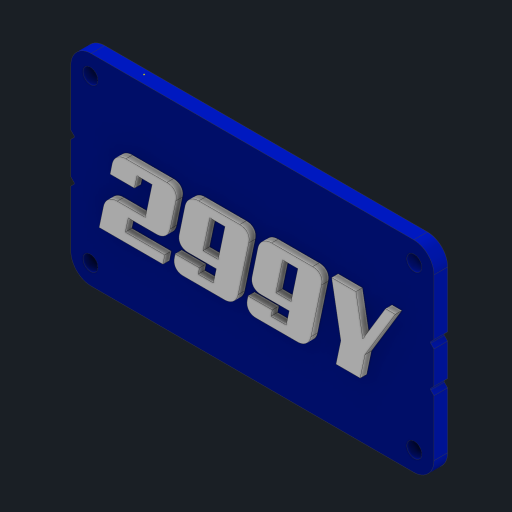
# Autodesk Inventor part: 299Y
Saved by Autodesk Inventor 2023 (Build 270158000, 158)
## iProperties
Created: 2023-05-30
Part Number: 299Y
Material: Generic
Document SubType Name: Modeling
Designer: reima
Density: 1 g/cm^3
Appearance: Default
Author: reima
Autodesk Inventor part; units mm, degrees
ref_plane "YZ Plane" through (0, 0, 0) normal (1, 0, 0) x (0, 1, 0)
ref_plane "XZ Plane" through (0, 0, 0) normal (0, 1, 0) x (-1, 0, 0)
ref_plane "XY Plane" through (0, 0, 0) normal (0, 0, 1) x (1, 0, 0)
sketch "Sketch1" plane through (0, 0, 0) normal (0, 0, 1) x (1, 0, 0)
  circle A0 centre (-16.8236, -8.8233) radius 2.1 projected
  circle A1 centre (84.7764, -8.8233) radius 2.1 projected
  circle A2 centre (84.7764, -59.6233) radius 2.1 projected
  circle A3 centre (-16.8236, -59.6233) radius 2.1 projected
  line L0 (-11.8121, -2.6233) -> (-16.8236, -2.6233) projected
  line L1 (84.7764, -65.7984) -> (79.7648, -65.7984) projected
  line L2 (90.9515, -41.9118) -> (90.9515, -51.9348) projected
  line L3 (-22.9988, -26.5348) -> (-22.9988, -16.5118) projected
  line L4 (-16.6488, -2.6233) -> (84.6015, -2.6233)
  line L5 (90.9515, -8.9733) -> (90.9515, -59.4484)
  line L6 (84.6015, -65.7984) -> (-16.6488, -65.7984)
  line L7 (-22.9988, -59.4484) -> (-22.9988, -8.9733)
  arc A4 (-16.6488, -2.6233) -> (-22.9988, -8.9733) centre (-16.6488, -8.9733) ccw
  arc A5 (-22.9988, -59.4484) -> (-16.6488, -65.7984) centre (-16.6488, -59.4484) ccw
  arc A6 (84.6015, -65.7984) -> (90.9515, -59.4484) centre (84.6015, -59.4484) ccw
  arc A7 (90.9515, -8.9733) -> (84.6015, -2.6233) centre (84.6015, -8.9733) ccw
  line L8 (-22.9988, -39.2857) -> (-21.9533, -40.3312)
  line L9 (-21.9533, -40.7802) -> (-22.9988, -41.8257)
  arc A8 (-21.9533, -40.7802) -> (-21.9533, -40.3312) centre (-22.1778, -40.5557) ccw
  line L10 (33.9764, -2.6233) -> (33.9764, -65.7984)
  line L11 (90.9515, -39.2857) -> (89.906, -40.3312)
  line L12 (89.906, -40.7802) -> (90.9515, -41.8257)
  arc A9 (89.906, -40.3312) -> (89.906, -40.7802) centre (90.1305, -40.5557) ccw
  point P0 (0, 0)
  point P1 (-22.9988, -2.6233)
  point P2 (90.9515, -65.7984)
  point P3 (90.9515, -2.6233)
  point P4 (-21.7288, -40.5557)
  dimension "d0" = 113.9502
  dimension "d1" = 63.1751
  dimension "d2" = 6.35
  dimension "d3" = 1.27
  dimension "d4" = 1.27
  dimension "d5" = 0.3175
  constraints: 18 end point, 12 point on circle, 10 point on line, 10 tangent, 6 centre point, 5 symmetric about line, 3 equal radius, 2 horizontal, 2 midpoint, 2 parallel, 2 perpendicular, 1 vertical, 1 other
  measures "d0" distance of point (-22.999, -2.623) point (90.951, -2.623)
  measures "d1" distance of point (90.951, -2.623) point (90.951, -65.798)
  measures "d2" radius of A4
  measures "d3" horizontal distance of L8.start point (-21.729, -40.556)
  measures "d4" horizontal distance of point (-21.729, -40.556) L9.end
  measures "d5" radius of A8
extrude "Extrusion1" add sketch "Sketch1" along normal blind 4.318 contours L4 L10 L6 A5 L7 L9 A8 L8 L3 A4 L0 | L4 A7 L5 L11 A9 L12 L2 A6 L1 L6 L10
sketch "Sketch2" plane through (0, 0, 4.318) normal (0, 0, 1) x (1, 0, 0)
  point P0 (0, 0)
sketch "Sketch3" plane through (0, 0, 4.318) normal (0, 0, 1) x (1, 0, 0)
  line L0 (-11.0608, -23.7053) -> (-1.734, -23.7053) construction
  line L1 (-1.734, -23.7053) -> (-1.734, -28.4261) construction
  line L2 (-1.734, -28.4261) -> (-11.0608, -28.4261) construction
  line L3 (-11.0608, -28.4261) -> (-11.0608, -23.7053) construction
  line L4 (84.6015, -2.6233) -> (-16.6488, -2.6233) construction
  line L5 (33.9764, -2.6233) -> (33.9764, -66.312) construction
  line L6 (-22.9988, -8.9733) -> (-22.9988, -39.2857) construction
  line L7 (-22.9988, -34.4676) -> (90.982, -34.4676) construction
  line L8 (-3.8427, -43.7165) -> (8.5485, -43.7165)
  line L9 (8.5485, -43.7165) -> (7.9543, -46.5653)
  line L10 (7.9543, -46.5653) -> (-12.0569, -46.5653)
  line L11 (-12.0569, -46.5653) -> (-10.6937, -40.1512)
  spline S0 degree 2 poles (-10.6937, -40.1512) (-10.3267, -38.5258) (-7.9498, -36.5684) (-6.3594, -36.5684) knots 0 0 0 1 2 2 2
  line L12 (-6.3594, -36.5684) -> (2.449, -36.5684)
  line L13 (2.449, -36.5684) -> (4.5637, -26.589)
  line L14 (4.5637, -26.589) -> (-0.19, -26.589)
  line L15 (-0.19, -26.589) -> (-0.994, -30.3641)
  line L16 (-0.994, -30.3641) -> (-8.614, -30.3641)
  line L17 (-8.614, -30.3641) -> (-7.9848, -27.2881)
  spline S1 degree 2 poles (-7.9848, -27.2881) (-7.6178, -25.6627) (-5.2234, -23.7053) (-3.6505, -23.7053) knots 0 0 0 1 2 2 2
  line L18 (-3.6505, -23.7053) -> (9.2126, -23.7053)
  spline S2 degree 2 poles (9.2126, -23.7053) (10.838, -23.7053) (12.3935, -25.6627) (12.0264, -27.2881) knots 0 0 0 1 2 2 2
  line L19 (12.0264, -27.2881) -> (10.2263, -35.8344)
  spline S3 degree 2 poles (10.2263, -35.8344) (9.8768, -37.4597) (7.4824, -39.4172) (5.892, -39.4172) knots 0 0 0 1 2 2 2
  line L20 (5.892, -39.4172) -> (-2.9164, -39.4172)
  line L21 (-2.9164, -39.4172) -> (-3.8427, -43.7165)
  spline S4 degree 2 poles (14.8752, -27.2881) (15.2422, -25.6627) (17.6366, -23.7053) (19.2095, -23.7053) knots 0 0 0 1 2 2 2
  line L22 (19.2095, -23.7053) -> (32.0726, -23.7053)
  spline S5 degree 2 poles (32.0726, -23.7053) (33.698, -23.7053) (35.2535, -25.6627) (34.8864, -27.2881) knots 0 0 0 1 2 2 2
  line L23 (34.8864, -27.2881) -> (31.5658, -42.9825)
  spline S6 degree 2 poles (31.5658, -42.9825) (31.1988, -44.6079) (28.8219, -46.5653) (27.2315, -46.5653) knots 0 0 0 1 2 2 2
  line L24 (27.2315, -46.5653) -> (14.3859, -46.5653)
  spline S7 degree 2 poles (14.3859, -46.5653) (12.7605, -46.5653) (11.24, -44.6079) (11.572, -42.9825) knots 0 0 0 1 2 2 2
  line L25 (11.572, -42.9825) -> (11.7992, -41.7941)
  line L26 (11.7992, -41.7941) -> (19.4192, -41.7941)
  line L27 (19.4192, -41.7941) -> (19.0173, -43.7165)
  line L28 (19.0173, -43.7165) -> (23.7885, -43.7165)
  line L29 (23.7885, -43.7165) -> (24.7148, -39.4172)
  line L30 (24.7148, -39.4172) -> (15.9064, -39.4172)
  spline S8 degree 2 poles (15.9064, -39.4172) (14.281, -39.4172) (12.7255, -37.4597) (13.0925, -35.8344) knots 0 0 0 1 2 2 2
  line L31 (13.0925, -35.8344) -> (14.8752, -27.2881)
  line L32 (22.67, -26.589) -> (20.5378, -36.5684)
  line L33 (20.5378, -36.5684) -> (25.309, -36.5684)
  line L34 (25.309, -36.5684) -> (27.4237, -26.589)
  line L35 (27.4237, -26.589) -> (22.67, -26.589)
  spline S9 degree 2 poles (37.7352, -27.2881) (38.1022, -25.6627) (40.4966, -23.7053) (42.0695, -23.7053) knots 0 0 0 1 2 2 2
  line L36 (42.0695, -23.7053) -> (54.9326, -23.7053)
  spline S10 degree 2 poles (54.9326, -23.7053) (56.558, -23.7053) (58.1135, -25.6627) (57.7464, -27.2881) knots 0 0 0 1 2 2 2
  line L37 (57.7464, -27.2881) -> (54.4258, -42.9825)
  spline S11 degree 2 poles (54.4258, -42.9825) (54.0588, -44.6079) (51.6819, -46.5653) (50.0915, -46.5653) knots 0 0 0 1 2 2 2
  line L38 (50.0915, -46.5653) -> (37.2459, -46.5653)
  spline S12 degree 2 poles (37.2459, -46.5653) (35.6205, -46.5653) (34.1, -44.6079) (34.432, -42.9825) knots 0 0 0 1 2 2 2
  line L39 (34.432, -42.9825) -> (34.6592, -41.7941)
  line L40 (34.6592, -41.7941) -> (42.2792, -41.7941)
  line L41 (42.2792, -41.7941) -> (41.8773, -43.7165)
  line L42 (41.8773, -43.7165) -> (46.6485, -43.7165)
  line L43 (46.6485, -43.7165) -> (47.5748, -39.4172)
  line L44 (47.5748, -39.4172) -> (38.7664, -39.4172)
  spline S13 degree 2 poles (38.7664, -39.4172) (37.141, -39.4172) (35.5855, -37.4597) (35.9525, -35.8344) knots 0 0 0 1 2 2 2
  line L45 (35.9525, -35.8344) -> (37.7352, -27.2881)
  line L46 (45.53, -26.589) -> (43.3978, -36.5684)
  line L47 (43.3978, -36.5684) -> (48.169, -36.5684)
  line L48 (48.169, -36.5684) -> (50.2837, -26.589)
  line L49 (50.2837, -26.589) -> (45.53, -26.589)
  line L50 (71.3611, -39.4172) -> (69.8406, -46.5653)
  line L51 (69.8406, -46.5653) -> (62.2555, -46.5653)
  line L52 (62.2555, -46.5653) -> (63.776, -39.4172)
  line L53 (63.776, -39.4172) -> (60.8923, -23.7053)
  line L54 (60.8923, -23.7053) -> (68.5123, -23.7053)
  line L55 (68.5123, -23.7053) -> (70.662, -35.5023)
  line L56 (70.662, -35.5023) -> (77.7926, -23.7053)
  line L57 (77.7926, -23.7053) -> (80.8686, -23.7053)
  line L58 (80.8686, -23.7053) -> (71.3611, -39.4172)
  point P0 (0, 0)
  point P1 (-11.0608, -26.0657)
  dimension "d8" = 11.938
  dimension "d11" = 21.082
  constraints: 4 end point, 2 midpoint, 1 perpendicular, 1 point on line, 1 vertical, 2 other
  measures "d8" distance from line of L6 point (-11.061, -26.066)
  measures "d11" distance between parallel lines of L4 L0
extrude "Extrusion3" add sketch "Sketch3" along normal blind 2.032
sketch "Sketch4" plane through (0, 0, 4.318) normal (0, 0, 1) x (1, 0, 0)
  line L0 (-22.9988, -39.2857) -> (-21.9533, -40.3312) projected
  line L1 (-21.9533, -40.7802) -> (-22.9988, -41.8257) projected
  arc A0 (-21.9533, -40.7802) -> (-21.9533, -40.3312) centre (-22.1778, -40.5557) ccw projected
  line L2 (90.9515, -41.8257) -> (89.906, -40.7802) projected
  arc A1 (89.906, -40.3312) -> (89.906, -40.7802) centre (90.1305, -40.5557) ccw projected
  line L3 (89.906, -40.3312) -> (90.9515, -39.2857) projected
  line L4 (-22.9988, -8.9733) -> (-22.9988, -39.2857) construction
  line L5 (-22.9988, -34.2082) -> (90.9515, -34.2082) construction
  line L6 (90.9515, -39.2857) -> (90.9515, -8.9733) construction
  line L7 (84.6015, -2.6233) -> (-16.6488, -2.6233) construction
  line L8 (-22.9988, -29.1307) -> (-21.9533, -28.0852)
  line L9 (-21.9533, -27.6362) -> (-22.9988, -26.5907)
  arc A2 (-21.9533, -28.0852) -> (-21.9533, -27.6362) centre (-22.1778, -27.8607) ccw
  line L10 (90.9515, -26.5907) -> (89.906, -27.6362)
  arc A3 (89.906, -27.6362) -> (89.906, -28.0852) centre (90.1305, -27.8607) ccw
  line L11 (89.906, -28.0852) -> (90.9515, -29.1307)
  line L12 (90.9515, -26.5907) -> (90.9515, -29.1307) construction
  line L13 (-22.9988, -26.5907) -> (-22.9988, -29.1307) construction
  line L14 (-22.9988, -26.5907) -> (-22.9988, -29.1307)
  line L15 (90.9515, -26.5907) -> (90.9515, -29.1307)
  point P0 (0, 0)
  dimension "d14" = 31.5849
  constraints: 18 end point, 10 symmetric about line, 4 point on circle, 4 point on line, 2 centre point, 2 parallel, 1 collinear, 1 horizontal, 2 other
  measures "d14" distance between parallel lines of L5 L7
extrude "Extrusion4" cut sketch "Sketch4" against normal through all
sketch "Sketch5" plane through (0, 0, 4.318) normal (0, 0, 1) x (1, 0, 0)
  circle A0 centre (-16.8236, -8.8233) radius 2.1 projected
  circle A1 centre (-16.8236, -8.8233) radius 2.3368
  circle A2 centre (84.7764, -8.8233) radius 2.1 projected
  circle A3 centre (84.7764, -59.6233) radius 2.1 projected
  circle A4 centre (-16.8236, -59.6233) radius 2.1 projected
  circle A5 centre (84.7764, -8.8233) radius 2.3368
  circle A6 centre (84.7764, -59.6233) radius 2.3368
  circle A7 centre (-16.8236, -59.6233) radius 2.3368
  point P0 (0, 0)
  dimension "d17" = 4.6736
  dimension "d18" = 4.6736
  dimension "d19" = 4.6736
  dimension "d20" = 4.6736
  constraints: 4 centre point, 4 coincident
  measures "d17" diameter of A1
  measures "d18" diameter of A5
  measures "d19" diameter of A6
  measures "d20" diameter of A7
extrude "Extrusion5" cut sketch "Sketch5" against normal blind 25.4
body "Solid1"
